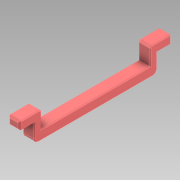
# Autodesk Inventor part: TrussCC_S1
Saved by Autodesk Inventor 2021 (Build 250183000, 183)
## iProperties
Created: 2021-02-11
Part Number: TrussCC_S1
Material: 一般
Document SubType Name: Modeling
Designer: kumagai
Density: 1 g/cm^3
Appearance: 滑らか - 赤
Author: kumagai
Autodesk Inventor part; units mm, degrees
ref_plane "YZ Plane" through (0, 0, 0) normal (1, 0, 0) x (0, 1, 0)
ref_plane "XZ Plane" through (0, 0, 0) normal (0, 1, 0) x (-1, 0, 0)
ref_plane "XY Plane" through (0, 0, 0) normal (0, 0, 1) x (1, 0, 0)
sketch "スケッチ1" plane through (0, 0, 0) normal (1, 0, 0) x (0, 1, 0)
  line L0 (-6.16, 0) -> (8.96, 0) projected
  line L1 (0, 43.4) -> (0, -43.4) projected
  line L2 (0, 22) -> (0, -22)
  line L3 (0, -22) -> (7.1, -22)
  line L4 (7.1, -22) -> (7.1, -31)
  line L5 (7.1, -31) -> (3.5, -31)
  line L6 (3.5, -31) -> (3.5, -25)
  line L7 (3.5, -25) -> (-4, -25)
  line L8 (-4, -25) -> (-4, 25)
  line L9 (-4, 25) -> (3.5, 25)
  line L10 (3.5, 25) -> (3.5, 31)
  line L11 (3.5, 31) -> (7.1, 31)
  line L12 (7.1, 31) -> (7.1, 22)
  line L13 (7.1, 22) -> (0, 22)
  point P0 (0, 0)
  dimension "d0" = 3.5
  dimension "d1" = 4
  dimension "d2" = 50
  dimension "d3" = 6
  dimension "d4" = 3
  dimension "d5" = 3.6
  constraints: 24 end point, 7 perpendicular, 4 point on line, 1 collinear, 1 horizontal, 1 parallel, 3 other
  measures "d0" distance between parallel lines of L1 L6
  measures "d1" distance between parallel lines of L8 L1
  measures "d2" distance between parallel lines of L7 L9
  measures "d3" distance between parallel lines of L11 L9
  measures "d4" distance between parallel lines of L13 L9
  measures "d5" distance between parallel lines of L10 L12
extrude "押し出し1" add sketch "スケッチ1" along normal mid plane 4.8
chamfer "面取り1" distance 0.8 angle 45 10 edges at (0, 7.1, 31) (0, 3.5, 31) (2.4, 5.3, 31) (-2.4, 5.3, 31) (2.4, 5.3, -31) (0, 7.1, -31) (-2.4, 5.3, -31) (0, 3.5, -31) (0, 7.1, 22) (0, 7.1, -22)
fillet "フィレット1" radius 2 2 edges at (0, -4, 25) (0, -4, -25)
chamfer "面取り2" distance 0.4 angle 45 28 edges at (2.4, -4, 0) (2.4, -3.4142, -24.4142) (2.4, 0.75, -25) (2.4, 3.5, -27.6) (2.4, -3.4142, 24.4142) (2.4, 0.75, 25) (2.4, 3.5, 27.6) (-2.4, 0.75, 25) (-2.4, -3.4142, 24.4142) (-2.4, 3.5, 27.6) (-2.4, -4, 0) (-2.4, -3.4142, -24.4142) (-2.4, 0.75, -25) (-2.4, 3.5, -27.6) (2.4, 0, 0) (-2.4, 0, 0) (2.4, 3.15, -22) (2.4, 6.7, -22.4) (2.4, 7.1, -26.5) (-2.4, 7.1, -26.5) (-2.4, 6.7, -22.4) (-2.4, 3.15, -22) (-2.4, 3.15, 22) (-2.4, 6.7, 22.4) (-2.4, 7.1, 26.5) (2.4, 7.1, 26.5) (2.4, 6.7, 22.4) (2.4, 3.15, 22)
